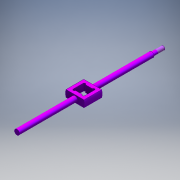
# Autodesk Inventor part: Asta pistone
Saved by Autodesk Inventor 2016 (Build 200138000, 138)
## iProperties
Created: 2016-11-28
Part Number: Asta pistone
Material: Generic
Document SubType Name: Modeling
Designer: Muhammad
Density: 1 g/cm^3
Appearance: Default
Author: Muhammad
Autodesk Inventor part; units mm, degrees
ref_plane "YZ Plane" through (0, 0, 0) normal (1, 0, 0) x (0, 1, 0)
ref_plane "XZ Plane" through (0, 0, 0) normal (0, 1, 0) x (-1, 0, 0)
ref_plane "XY Plane" through (0, 0, 0) normal (0, 0, 1) x (1, 0, 0)
sketch "Sketch1" plane through (0, 0, 0) normal (0, 1, 0) x (-1, 0, 0)
  line L0 (12.5, 0) -> (12.5, 4.5) construction
  line L1 (12.5, 4.5) -> (12.5, -4.5) construction
  line L2 (11.6619, 4.5) -> (-11.6619, 4.5)
  line L3 (11.6619, -4.5) -> (-11.6619, -4.5)
  arc A0 (11.6619, -4.5) -> (11.6619, 4.5) centre (0, 0) ccw
  arc A1 (-11.6619, 4.5) -> (-11.6619, -4.5) centre (0, 0) ccw
  dimension "d1" = 4.5
  dimension "d2" = 9
  constraints: 8 end point, 5 point on circle, 2 centre point, 1 coincident, 1 horizontal, 1 parallel, 1 point on line, 1 tangent, 1 vertical
  measures "d1" distance of L0.start L0.end
  measures "d2" distance of L0.end L1.end
extrude "Extrusion1" add sketch "Sketch1" along normal mid plane 23
sketch "Sketch2" plane through (-11.6619, -11.5, 4.5) normal (0, 0, 1) x (1, 0, 0)
  line L0 (7.1619, 5) -> (16.1619, 5)
  line L1 (19.1619, 5) -> (19.1619, 18)
  line L2 (4.1619, 18) -> (4.1619, 5)
  line L3 (11.6619, 11.5) -> (19.1619, 18) construction
  line L4 (19.1619, 5) -> (11.6619, 11.5) construction
  line L5 (4.1619, 5) -> (5.6619, 5) construction
  arc A0 (4.1619, 5) -> (7.1619, 5) centre (5.6619, 5) ccw
  line L6 (4.1619, 18) -> (5.6619, 18) construction
  arc A1 (7.1619, 18) -> (4.1619, 18) centre (5.6619, 18) ccw
  line L7 (19.1619, 5) -> (17.6619, 5) construction
  arc A2 (16.1619, 5) -> (19.1619, 5) centre (17.6619, 5) ccw
  arc A3 (17.6619, 6.5) -> (17.4487, 6.4848) centre (17.6619, 5) ccw
  arc A4 (19.1619, 18) -> (16.1619, 18) centre (17.6619, 18) ccw
  arc A5 (17.4487, 16.5152) -> (17.6619, 16.5) centre (17.6619, 18) ccw
  line L8 (16.1619, 18) -> (7.1619, 18)
  dimension "d8" = 1.5
  constraints: 18 end point, 12 point on circle, 6 centre point, 5 point on line, 3 coincident, 2 parallel, 1 horizontal, 1 perpendicular
  measures "d8" distance of L7.end L1.start
extrude "Extrusion2" cut sketch "Sketch2" against normal through all
sketch "Sketch3" plane through (0, -11.5, 0) normal (0, -1, 0) x (1, 0, 0)
  circle A0 centre (0, 0) radius 3.35
  dimension "d11" = 6.7
  constraints: 1 centre point, 1 coincident
  measures "d11" diameter of A0
extrude "Extrusion3" add sketch "Sketch3" along normal blind 75.5
sketch "Sketch4" plane through (0, 11.5, 0) normal (0, 1, 0) x (1, 0, 0)
  circle A0 centre (0, 0) radius 3.35
  dimension "d14" = 6.7
  constraints: 1 centre point, 1 coincident
  measures "d14" diameter of A0
extrude "Extrusion4" add sketch "Sketch4" along normal blind 76.5
sketch "Sketch5" plane through (0, 88, 0) normal (0, 1, 0) x (1, 0, 0)
  circle A0 centre (0, 0) radius 2.5
  dimension "d17" = 5
  constraints: 1 centre point, 1 coincident
  measures "d17" diameter of A0
extrude "Extrusion5" add sketch "Sketch5" along normal blind 15
thread "Thread1" size "M5x0.8" class "6g" standard "ANSI Metric M Profile" length 9
body "Solid1"
